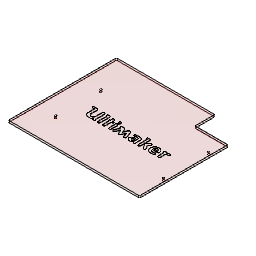
PCBCover_v9 (Autodesk Fusion 360 design; units mm, degrees)
Autodesk Fusion 360 part; units mm, degrees
note: some values were not read from the file. Set by a fixed rule: which sketch regions a step uses.
(part 1 of 5)
sketch "Sketch1" plane through (0, 0, 0) normal (0, 0, 1) x (1, 0, 0) in component "PCB Cover"
  line L0 (0, 0) -> (200, 0)
  line L1 (200, 0) -> (200, 165)
  line L2 (200, 165) -> (0, 165)
  line L3 (0, 165) -> (0, 0)
  line L4 (0, 42) -> (200, 42) construction
  line L5 (0, 111) -> (200, 111) construction
  line L6 (195, 165) -> (195, 0) construction
  line L7 (30, 165) -> (30, 0) construction
  circle A0 centre (30, 111) radius 1.5
  circle A1 centre (30, 42) radius 1.5
  circle A2 centre (195, 111) radius 1.5
  circle A3 centre (195, 42) radius 1.5
  line L8 (150, 165) -> (150, 135)
  line L9 (150, 135) -> (200, 135)
  dimension "d1_1" = 200
  dimension "d2_1" = 165
  dimension "d3_1" = 42
  dimension "d4_1" = 69
  dimension "d5_1" = 5
  dimension "d6_1" = 165
  dimension "d8_1" = 3
  dimension "d9_1" = 3
  dimension "d10_1" = 3
  dimension "d11_1" = 3
  dimension "d19" = 50
  dimension "d20" = 30
  constraint horizontal L0
  constraint vertical L1
  constraint horizontal L2
  constraint vertical L3
  constraint coincident L0.start L3.end
  constraint coincident L3 L4.start
  constraint coincident L1 L4.end
  constraint perpendicular L1 L4
  constraint coincident L3 L5.start
  constraint coincident L1 L5.end
  constraint perpendicular L1 L5
  constraint coincident L2 L6.start
  constraint coincident L0 L6.end
  constraint perpendicular L0 L6
  constraint coincident L2 L7.start
  constraint coincident L0 L7.end
  constraint perpendicular L0 L7
  constraint coincident L7 A0.centre
  constraint coincident L5 A0.centre
  constraint coincident L4 A1.centre
  constraint coincident L7 A1.centre
  constraint coincident L5 A2.centre
  constraint coincident L6 A2.centre
  constraint coincident L6 A3.centre
  constraint coincident L4 A3.centre
  constraint coincident L2 L8.start
  constraint perpendicular L2 L8
  constraint coincident L1 L9.end
  constraint perpendicular L1 L9
  measures "d1_1" distance of L1 L3
  measures "d2_1" distance of L0 L2
  measures "d3_1" distance of L0 L4
  measures "d4_1" distance of L4 L5
  measures "d5_1" distance of L1 L6
  measures "d6_1" distance of L6 L7
  measures "d8_1" diameter of A0
  measures "d9_1" diameter of A2
  measures "d10_1" diameter of A1
  measures "d11_1" diameter of A3
  measures "d19" distance of L1 L8
  measures "d20" distance of L2 L9
extrude "Extrude1" add sketch "Sketch1" along normal blind 3 contours L0 L1 L2 L3 L8 L9 in component "PCB Cover"
fillet "Fillet1" radius 1 6 edges at (0, 0, 1.5) (200, 0, 1.5) (0, 165, 1.5) (150, 165, 1.5) (150, 135, 1.5) (200, 135, 1.5) in component "PCB Cover"
sketch "Sketch3" plane through (0, 0, 3) normal (0, 0, 1) x (-1, 0, 0) in component "PCB Cover"
  arc A0 (-1, -165) -> (0, -164) centre (-1, -164) ccw
  line L0 (0, -164) -> (0, -1)
  arc A1 (0, -1) -> (-1, 0) centre (-1, -1) ccw
  line L1 (-1, 0) -> (-199, 0)
  arc A2 (-199, 0) -> (-200, -1) centre (-199, -1) ccw
  line L2 (-200, -1) -> (-200, -134)
  line L3 (-149, -165) -> (-1, -165)
  circle A3 centre (-195, -111) radius 1.5
  circle A4 centre (-195, -42) radius 1.5
  circle A5 centre (-30, -42) radius 1.5
  circle A6 centre (-30, -111) radius 1.5
  line L4 (-68.801, -83.1029) -> (-68.7045, -83.0443)
  line L5 (-134.3507, -66.6361) -> (-134.3896, -66.8178)
  line L6 (-62.8852, -66.514) -> (-62.9029, -66.3979)
  line L7 (-121.6987, -75.685) -> (-122.1036, -75.6545)
  line L8 (-118.5, -69.5598) -> (-118.5454, -69.7228)
  line L9 (-141.8993, -76.7576) -> (-141.9093, -76.9708)
  line L10 (-88.7696, -78.5031) -> (-88.9694, -78.4589)
  line L11 (-89.0089, -83.178) -> (-89.1669, -83.1019)
  line L12 (-112.6227, -67.3536) -> (-112.6072, -67.5226)
  line L13 (-88.9694, -78.4589) -> (-89.1489, -78.3988)
  line L14 (-122.1036, -75.6545) -> (-122.294, -75.6283)
  line L15 (-129.3707, -81.8373) -> (-129.3995, -81.725)
  line L16 (-79.0047, -82.0756) -> (-78.8216, -82.0548)
  line L17 (-130.9813, -66.8178) -> (-131.0201, -66.6361)
  line L18 (-62.9029, -66.3979) -> (-62.9317, -66.2857)
  line L19 (-93.4282, -77.1585) -> (-93.4342, -77.0387)
  line L20 (-141.7632, -77.5869) -> (-141.6868, -77.7243)
  line L21 (-129.7727, -81.1699) -> (-129.8628, -81.1025)
  line L22 (-90.112, -81.5125) -> (-90.103, -81.3276)
  line L23 (-76.2839, -77.4043) -> (-76.2551, -77.2923)
  line L24 (-69.6946, -66.6366) -> (-69.7482, -66.468)
  line L25 (-118.4981, -68.9082) -> (-118.4726, -69.0494)
  line L26 (-52.3978, -83.2329) -> (-52.2486, -83.2445)
  line L27 (-108.4802, -77.8696) -> (-108.3282, -77.9669)
  line L28 (-73.0643, -66.8183) -> (-73.088, -67.0129)
  line L29 (-109.5517, -66.2313) -> (-109.6365, -66.1302)
  line L30 (-98.0467, -78.3289) -> (-94.5986, -78.3289)
  line L31 (-117.5374, -72.5382) -> (-117.3342, -72.4627)
  line L32 (-54.1692, -81.8436) -> (-54.1178, -82.0155)
  line L33 (-120.6684, -72.9315) -> (-120.5332, -72.9709)
  line L34 (-156.7744, -71.3956) -> (-156.9307, -71.4261)
  line L35 (-135.3769, -72.8016) -> (-135.4061, -72.608)
  line L36 (-102.0665, -65.767) -> (-102.0887, -65.7551)
  line L37 (-101.3094, -66.4135) -> (-101.3514, -66.355)
  line L38 (-130.1691, -83.1912) -> (-130.0616, -83.1518)
  line L39 (-77.8285, -81.5268) -> (-77.7337, -81.3976)
  line L40 (-68.5313, -81.246) -> (-68.6144, -81.1705)
  line L41 (-134.1478, -82.5385) -> (-134.053, -82.6678)
  line L42 (-93.9443, -76.1877) -> (-94.0408, -76.1291)
  line L43 (-131.425, -65.9244) -> (-131.5448, -65.8219)
  line L44 (-65.2234, -72.2146) -> (-65.2234, -81.2746)
  line L45 (-109.0017, -77.3755) -> (-108.8856, -77.5138)
  line L46 (-98.1858, -78.3189) -> (-98.0467, -78.3289)
  line L47 (-73.0304, -82.0535) -> (-72.9802, -82.2175)
  line L48 (-121.4694, -71.7956) -> (-121.4581, -71.9616)
  line L49 (-133.6942, -65.7328) -> (-133.8257, -65.8219)
  line L50 (-70.2196, -65.8224) -> (-70.3511, -65.7333)
  line L51 (-59.741, -68.9094) -> (-59.5923, -68.8427)
  line L52 (-104.0125, -66.1757) -> (-104.086, -66.2611)
  line L53 (-86.5793, -82.05) -> (-86.64, -82.2161)
  line L54 (-93.6955, -76.4137) -> (-93.7711, -76.3306)
  line L55 (-53.0837, -83.0778) -> (-52.9126, -83.1337)
  line L56 (-110.7765, -65.5715) -> (-110.908, -65.5665)
  line L57 (-62.6523, -83.1446) -> (-62.4675, -83.0838)
  line L58 (-87.1608, -65.7896) -> (-87.0368, -65.8914)
  line L59 (-129.3707, -82.3092) -> (-129.353, -82.193)
  line L60 (-99.6212, -77.9746) -> (-99.4654, -78.0571)
  line L61 (-132.3759, -83.2437) -> (-130.5171, -83.2437)
  line L62 (-87.2947, -80.0143) -> (-87.1556, -80.1182)
  line L63 (-135.417, -73.5132) -> (-135.39, -73.3534)
  line L64 (-78.3302, -81.9099) -> (-78.1873, -81.8343)
  line L65 (-166.0715, -78.5875) -> (-165.9299, -78.5695)
  line L66 (-86.6139, -77.3087) -> (-86.6505, -77.4665)
  line L67 (-102.4573, -65.6498) -> (-102.6019, -65.6294)
  line L68 (-88.1205, -79.7153) -> (-87.941, -79.7427)
  line L69 (-92.9842, -66.7) -> (-93.0475, -66.548)
  line L70 (-54.9561, -69.5643) -> (-54.859, -69.6851)
  line L71 (-61.6272, -82.4034) -> (-61.5365, -82.243)
  line L72 (-61.4612, -82.0706) -> (-61.4018, -81.887)
  line L73 (-135.5106, -72.2342) -> (-135.5805, -72.0567)
  line L74 (-110.2717, -65.6893) -> (-110.3937, -65.6458)
  line L75 (-87.3025, -78.3238) -> (-87.4627, -78.3988)
  line L76 (-73.0668, -81.8773) -> (-73.0304, -82.0535)
  line L77 (-98.4083, -78.3) -> (-98.3201, -78.293)
  line L78 (-86.7617, -77.7607) -> (-86.8381, -77.8951)
  line L79 (-86.8381, -77.8951) -> (-86.9295, -78.0196)
  line L80 (-109.7282, -66.0365) -> (-109.8263, -65.9506)
  line L81 (-69.0109, -80.9558) -> (-69.1231, -80.927)
  line L82 (-90.0311, -82.05) -> (-90.0756, -81.8768)
  line L83 (-135.3726, -73.1817) -> (-135.3666, -72.9978)
  line L84 (-69.624, -80.9033) -> (-69.624, -67.2204)
  line L85 (-138.937, -77.8736) -> (-135.9197, -74.5208)
  line L86 (-88.7696, -65.5214) -> (-88.5487, -65.4942)
  line L87 (-105.5984, -77.78) -> (-105.4645, -77.6658)
  line L88 (-129.4388, -81.6175) -> (-129.4881, -81.5151)
  line L89 (-93.0475, -66.548) -> (-93.125, -66.4027)
  line L90 (-50.3366, -72.2147) -> (-50.3446, -71.781)
  line L91 (-59.1098, -68.6816) -> (-58.937, -68.6408)
  line L92 (-76.4986, -77.8006) -> (-76.4312, -77.7105)
  line L93 (-112.2905, -66.2655) -> (-112.3816, -66.403)
  line L94 (-101.743, -65.9554) -> (-101.7987, -65.9127)
  line L95 (-55.5404, -69.0628) -> (-55.4106, -69.1495)
  line L96 (-166.2167, -78.5935) -> (-166.0715, -78.5875)
  line L97 (-139.2218, -78.1381) -> (-139.075, -78.0114)
  line L98 (-88.063, -65.4942) -> (-87.842, -65.5214)
  line L99 (-50.3446, -71.781) -> (-50.3698, -71.3623)
  line L100 (-117.2991, -65.7945) -> (-117.4702, -65.7305)
  line L101 (-135.7422, -74.2993) -> (-135.641, -74.1334)
  line L102 (-108.7595, -77.6426) -> (-108.6242, -77.7613)
  line L103 (-168.7068, -75.6501) -> (-168.8644, -75.6788)
  line L104 (-89.0089, -79.8479) -> (-88.8429, -79.7872)
  line L105 (-66.3009, -66.1782) -> (-66.3403, -66.2857)
  line L106 (-46.1692, -81.9544) -> (-46.187, -81.8381)
  line L107 (-134.3896, -66.8178) -> (-134.4133, -67.0124)
  line L108 (-80.6588, -81.3976) -> (-80.5641, -81.5268)
  line L109 (-65.5702, -67.7507) -> (-65.458, -67.7795)
  line L110 (-101.9294, -65.8342) -> (-102.0665, -65.767)
  line L111 (-118.4726, -69.0494) -> (-118.4636, -69.1947)
  line L112 (-105.1182, -77.267) -> (-105.0233, -77.1168)
  line L113 (-46.5062, -81.2463) -> (-46.5893, -81.1708)
  line L114 (-109.2926, -66.7055) -> (-109.3443, -66.577)
  line L115 (-103.256, -65.7012) -> (-103.3662, -65.7391)
  line L116 (-73.096, -67.2204) -> (-73.096, -81.4885)
  line L117 (-46.5062, -82.9017) -> (-46.4306, -82.8186)
  line L118 (-65.7801, -67.6622) -> (-65.6778, -67.7114)
  line L119 (-66.2516, -67.1913) -> (-66.1929, -67.2877)
  line L120 (-86.5744, -67.0481) -> (-86.5694, -67.2203)
  line L121 (-76.4312, -77.7105) -> (-76.3726, -77.614)
  line L122 (-76.2551, -77.2923) -> (-76.2374, -77.1762)
  line L123 (-133.2339, -83.1617) -> (-133.0602, -83.1964)
  line L124 (-94.9876, -65.6109) -> (-95.1128, -65.6452)
  line L125 (-72.8225, -66.17) -> (-72.904, -66.3124)
  line L126 (-62.2947, -83.007) -> (-62.1343, -82.9148)
  line L127 (-80.4565, -65.8538) -> (-80.564, -65.9697)
  line L128 (-80.3368, -65.7513) -> (-80.4565, -65.8538)
  line L129 (-68.7045, -83.0443) -> (-68.6144, -82.9769)
  line L130 (-61.2891, -71.2837) -> (-61.2627, -71.0913)
  line L131 (-103.4191, -65.7552) -> (-103.4417, -65.7676)
  line L132 (-129.7727, -82.9765) -> (-129.6896, -82.9009)
  line L133 (-89.6998, -80.3631) -> (-89.5832, -80.2348)
  line L134 (-119.1134, -68.0951) -> (-118.9816, -68.1873)
  line L135 (-110.0394, -65.803) -> (-110.1534, -65.7418)
  line L136 (-107.288, -78.2938) -> (-107.0996, -78.3008)
  line L137 (-66.1929, -67.2877) -> (-66.1255, -67.3777)
  line L138 (-107.0926, -78.3) -> (-106.9084, -78.293)
  line L139 (-79.3885, -82.0756) -> (-79.1967, -82.0826)
  line L140 (-61.3587, -81.6928) -> (-61.3325, -81.4884)
  line L141 (-95.5765, -65.8721) -> (-95.6805, -65.95)
  line L142 (-86.6995, -66.407) -> (-86.6505, -66.5581)
  line L143 (-56.1554, -65.4904) -> (-56.5461, -65.4465)
  line L144 (-64.0494, -65.4636) -> (-65.222, -65.4636)
  line L145 (-79.9088, -65.5246) -> (-80.0624, -65.5866)
  line L146 (-65.8766, -65.6634) -> (-65.9667, -65.7308)
  line L147 (-66.3868, -66.7532) -> (-66.3691, -66.8694)
  line L148 (-80.5641, -81.5268) -> (-80.4566, -81.6427)
  line L149 (-80.8617, -80.931) -> (-80.8081, -81.0996)
  line L150 (-73.088, -67.0129) -> (-73.096, -67.2204)
  line L151 (-118.8637, -68.2887) -> (-118.7602, -68.3986)
  line L152 (-86.5074, -81.3276) -> (-86.4984, -81.5125)
  line L153 (-93.4519, -76.9224) -> (-93.4808, -76.8102)
  line L154 (-79.1967, -82.0826) -> (-79.0047, -82.0756)
  line L155 (-68.2409, -81.7256) -> (-68.2803, -81.618)
  line L156 (-136.1478, -71.1145) -> (-136.2972, -70.9305)
  line L157 (-129.6896, -81.2454) -> (-129.7727, -81.1699)
  line L158 (-78.8213, -65.4417) -> (-79.0043, -65.4208)
  line L159 (-101.7987, -65.9127) -> (-101.9294, -65.8342)
  line L160 (-93.9443, -78.129) -> (-93.8542, -78.0616)
  line L161 (-133.6942, -82.9756) -> (-133.5514, -83.0512)
  line L162 (-141.8251, -76.4251) -> (-141.8708, -76.5779)
  line L163 (-157.3994, -71.6624) -> (-157.4807, -71.7542)
  line L164 (-116.1043, -71.7474) -> (-115.9599, -71.6151)
  line L165 (-80.8617, -66.5655) -> (-80.9006, -66.7472)
  line L166 (-76.3233, -76.6007) -> (-76.3726, -76.4984)
  line L167 (-94.479, -78.3229) -> (-94.3628, -78.3051)
  line L168 (-140.2687, -78.5396) -> (-140.0758, -78.5266)
  line L169 (-55.9677, -68.8427) -> (-55.8191, -68.9094)
  line L170 (-80.9323, -78.2305) -> (-80.9323, -80.3472)
  line L171 (-109.4051, -66.455) -> (-109.4744, -66.3396)
  line L172 (-86.5348, -81.8768) -> (-86.5793, -82.05)
  line L173 (-118.5454, -69.7228) -> (-118.6087, -69.8735)
  line L174 (-159.5765, -77.2694) -> (-159.5942, -77.1532)
  line L175 (-94.8598, -65.586) -> (-94.9876, -65.6109)
  line L176 (-135.8309, -74.4188) -> (-135.7422, -74.2993)
  line L177 (-141.1482, -65.4851) -> (-141.3194, -65.4941)
  line L178 (-72.9166, -82.3692) -> (-72.8402, -82.5087)
  line L179 (-160.5044, -78.5352) -> (-160.3923, -78.5064)
  line L180 (-110.3937, -65.6458) -> (-110.5188, -65.6115)
  line L181 (-63.2738, -83.2247) -> (-63.056, -83.2157)
  line L182 (-165.6589, -78.5) -> (-165.5305, -78.4495)
  line L183 (-126.9226, -75.2022) -> (-126.9006, -75.4218)
  line L184 (-165.5305, -78.4495) -> (-165.4074, -78.3891)
  line L185 (-65.6778, -67.7114) -> (-65.5702, -67.7507)
  line L186 (-62.9711, -66.1782) -> (-63.0204, -66.076)
  line L187 (-76.3233, -77.5118) -> (-76.2839, -77.4043)
  line L188 (-59.4375, -68.7825) -> (-59.2767, -68.7288)
  line L189 (-80.9243, -66.9418) -> (-80.9323, -67.1493)
  line L190 (-59.6322, -65.5243) -> (-59.9762, -65.5837)
  line L191 (-120.4347, -70.8642) -> (-120.6989, -70.9072)
  line L192 (-106.9084, -78.293) -> (-106.7273, -78.2719)
  line L193 (-140.1409, -65.7466) -> (-140.2391, -65.691)
  line L194 (-83.5412, -77.2401) -> (-83.5221, -77.3781)
  line L195 (-161.4459, -66.1697) -> (-161.5406, -66.0405)
  line L196 (-89.912, -77.6175) -> (-89.961, -77.4665)
  line L197 (-123.9451, -66.3953) -> (-124.0398, -66.2386)
  line L198 (-118.9041, -70.2565) -> (-119.0371, -70.363)
  line L199 (-102.3649, -65.6702) -> (-102.4573, -65.6498)
  line L200 (-127.2707, -67.0128) -> (-127.2303, -67.206)
  line L201 (-122.801, -75.494) -> (-122.9443, -75.4272)
  line L202 (-95.3531, -65.7412) -> (-95.4672, -65.8024)
  line L203 (-148.3368, -72.1199) -> (-148.3504, -72.4808)
  line L204 (-88.5487, -65.4942) -> (-88.3059, -65.4852)
  line L205 (-142.7808, -67.0086) -> (-142.7888, -67.1725)
  line L206 (-54.237, -81.2746) -> (-54.229, -81.4727)
  line L207 (-156.082, -76.7687) -> (-155.8755, -76.964)
  line L208 (-131.0201, -66.6361) -> (-131.0736, -66.4674)
  line L209 (-118.5979, -68.6408) -> (-118.54, -68.7717)
  line L210 (-72.9718, -66.468) -> (-73.0254, -66.6366)
  line L211 (-83.1465, -77.9726) -> (-83.0413, -78.0357)
  line L212 (-140.5788, -65.5579) -> (-140.708, -65.5271)
  line L213 (-160.7403, -76.2193) -> (-161.1724, -76.2193)
  line L214 (-163.2831, -65.5128) -> (-163.4568, -65.5474)
  line L215 (-159.6623, -77.8448) -> (-159.623, -77.7373)
  line L216 (-125.5222, -77.3626) -> (-125.317, -77.4711)
  line L217 (-103.4417, -65.7676) -> (-103.5785, -65.8343)
  line L218 (-72.7513, -82.6359) -> (-72.6504, -82.7506)
  line L219 (-80.9006, -66.7472) -> (-80.9243, -66.9418)
  line L220 (-107.0996, -78.3008) -> (-107.0926, -78.3)
  line L221 (-131.1414, -66.3118) -> (-131.2229, -66.1694)
  line L222 (-159.623, -77.7373) -> (-159.5942, -77.6251)
  line L223 (-115.5046, -67.2364) -> (-115.6051, -67.0878)
  line L224 (-105.0233, -77.1168) -> (-104.9397, -76.9586)
  line L225 (-69.0109, -83.1916) -> (-68.9034, -83.1522)
  line L226 (-87.4437, -83.1019) -> (-87.6017, -83.178)
  line L227 (-129.8628, -81.1025) -> (-129.9593, -81.0439)
  line L228 (-93.3205, -66.1366) -> (-93.4375, -66.0181)
  line L229 (-61.7328, -82.5514) -> (-61.6272, -82.4034)
  line L230 (-95.1128, -65.6452) -> (-95.2348, -65.6887)
  line L231 (-92.9022, -67.0198) -> (-92.9356, -66.8576)
  line L232 (-65.3418, -67.7972) -> (-65.2235, -67.8035)
  line L233 (-125.4473, -65.4949) -> (-125.7165, -65.4841)
  line L234 (-89.8498, -77.7607) -> (-89.912, -77.6175)
  line L235 (-135.4521, -73.6609) -> (-135.417, -73.5132)
  line L236 (-54.859, -69.6851) -> (-54.7687, -69.813)
  line L237 (-80.8081, -81.0996) -> (-80.7403, -81.2552)
  line L238 (-159.623, -77.0411) -> (-159.6623, -76.9336)
  line L239 (-141.7635, -76.2923) -> (-141.8251, -76.4251)
  line L240 (-53.5344, -82.8302) -> (-53.395, -82.9256)
  line L241 (-142.3164, -65.9988) -> (-142.4212, -66.1208)
  line L242 (-87.6017, -83.178) -> (-87.7677, -83.2388)
  line L243 (-145.3418, -69.2555) -> (-145.4536, -68.9872)
  line L244 (-101.1722, -66.6714) -> (-101.2359, -66.5385)
  line L245 (-94.0408, -78.1876) -> (-93.9443, -78.129)
  line L246 (-116.2139, -66.4357) -> (-116.3544, -66.3241)
  line L247 (-134.4213, -81.4877) -> (-134.4133, -81.6953)
  line L248 (-54.0527, -82.1779) -> (-53.9742, -82.3302)
  line L249 (-159.5765, -77.5088) -> (-159.5705, -77.3891)
  line L250 (-87.0272, -80.2348) -> (-86.9106, -80.3631)
  line L251 (-106.7273, -78.2719) -> (-106.5499, -78.2376)
  line L252 (-120.8684, -65.7284) -> (-121.1733, -65.8221)
  line L253 (-46.5893, -82.9773) -> (-46.5062, -82.9017)
  line L254 (-145.8673, -68.2144) -> (-146.032, -67.9697)
  line L255 (-76.3726, -77.614) -> (-76.3233, -77.5118)
  line L256 (-132.6853, -65.4846) -> (-132.8771, -65.4916)
  line L257 (-72.0727, -65.5958) -> (-72.2263, -65.6578)
  line L258 (-114.9918, -69.0276) -> (-114.9978, -68.8249)
  line L259 (-64.2526, -83.007) -> (-64.0798, -83.0838)
  line L260 (-58.1882, -68.5413) -> (-57.78, -68.5289)
  line L261 (-89.961, -77.4665) -> (-89.9976, -77.3087)
  line L262 (-129.5467, -81.4186) -> (-129.6141, -81.3285)
  line L263 (-55.1702, -69.3433) -> (-55.0598, -69.4503)
  line L264 (-134.4213, -67.22) -> (-134.4213, -69.8591)
  line L265 (-119.5881, -67.881) -> (-119.417, -67.9412)
  line L266 (-104.1992, -66.4149) -> (-104.2726, -66.5393)
  line L267 (-159.996, -78.2921) -> (-159.9129, -78.2166)
  line L268 (-83.5412, -76.9402) -> (-83.5472, -77.0903)
  line L269 (-63.056, -83.2157) -> (-62.8487, -83.1888)
  line L270 (-54.2713, -71.2837) -> (-54.2524, -71.4835)
  line L271 (-83.3207, -77.8168) -> (-83.2396, -77.8997)
  line L272 (-164.9783, -78.0585) -> (-164.8891, -77.9561)
  line L273 (-77.936, -81.6427) -> (-77.8285, -81.5268)
  line L274 (-164.4235, -77.7499) -> (-164.3546, -77.8655)
  line L275 (-80.564, -65.9697) -> (-80.6588, -66.0989)
  line L276 (-161.1724, -76.2193) -> (-161.1724, -67.2203)
  line L277 (-163.2193, -78.5212) -> (-163.0667, -78.5355)
  line L278 (-119.0371, -70.363) -> (-119.1872, -70.4597)
  line L279 (-130.0616, -83.1518) -> (-129.9593, -83.1025)
  line L280 (-80.2054, -81.8343) -> (-80.0626, -81.9099)
  line L281 (-119.1872, -70.4597) -> (-119.354, -70.5472)
  line L282 (-127.1583, -66.2762) -> (-127.213, -66.401)
  line L283 (-107.8316, -78.1881) -> (-107.6547, -78.2368)
  line L284 (-157.4807, -71.7542) -> (-157.549, -71.8607)
  line L285 (-161.1724, -67.2203) -> (-161.1804, -67.0127)
  line L286 (-46.3632, -81.4195) -> (-46.4306, -81.3294)
  line L287 (-93.8542, -76.2551) -> (-93.9443, -76.1877)
  line L288 (-46.6794, -83.0447) -> (-46.5893, -82.9773)
  line L289 (-146.6097, -67.2837) -> (-146.8308, -67.0731)
  line L290 (-99.3035, -78.1282) -> (-99.1359, -78.1876)
  line L291 (-46.1632, -82.0741) -> (-46.1692, -81.9544)
  line L292 (-83.2396, -77.8997) -> (-83.1465, -77.9726)
  line L293 (-79.909, -81.9719) -> (-79.7451, -82.0202)
  line L294 (-135.9197, -74.5208) -> (-135.8309, -74.4188)
  line L295 (-164.808, -77.8468) -> (-164.7355, -77.7311)
  line L296 (-61.2576, -65.9312) -> (-61.5536, -66.0458)
  line L297 (-102.7545, -71.7649) -> (-100.6403, -76.7941)
  line L298 (-89.9976, -77.3087) -> (-90.0226, -77.145)
  line L299 (-103.3662, -65.7391) -> (-103.4191, -65.7552)
  line L300 (-133.9455, -82.7838) -> (-133.8257, -82.8864)
  line L301 (-65.2235, -67.8035) -> (-65.2215, -71.648)
  line L302 (-161.3644, -66.3121) -> (-161.4459, -66.1697)
  line L303 (-94.5986, -78.3289) -> (-94.479, -78.3229)
  line L304 (-68.1943, -81.9542) -> (-68.2121, -81.8379)
  line L305 (-68.9034, -80.9952) -> (-69.0109, -80.9558)
  line L306 (-82.9243, -78.0894) -> (-82.7955, -78.134)
  line L307 (-94.3628, -76.0117) -> (-94.479, -75.994)
  line L308 (-160.1826, -78.4179) -> (-160.0861, -78.3594)
  line L309 (-103.7091, -65.9129) -> (-103.7659, -65.9563)
  line L310 (-164.5739, -66.6363) -> (-164.6128, -66.8181)
  line L311 (-164.6183, -77.4824) -> (-164.5745, -77.3505)
  line L312 (-65.458, -65.4873) -> (-65.5702, -65.5161)
  line L313 (-79.5712, -65.4417) -> (-79.7449, -65.4763)
  line L314 (-122.1871, -78.2057) -> (-121.4511, -78.2582)
  line L315 (-94.1431, -78.2369) -> (-94.0408, -78.1876)
  line L316 (-83.0413, -78.0357) -> (-82.9243, -78.0894)
  line L317 (-151.4448, -78.5402) -> (-151.064, -78.5322)
  line L318 (-164.6445, -74.2229) -> (-166.4853, -75.6143)
  line L319 (-80.9323, -80.3472) -> (-80.9243, -80.5547)
  line L320 (-163.6208, -65.5957) -> (-163.7744, -65.6576)
  line L321 (-100.1696, -77.5402) -> (-100.045, -77.6636)
  line L322 (-105.8898, -77.9776) -> (-105.7403, -77.8841)
  line L323 (-53.9742, -82.3302) -> (-53.8827, -82.4721)
  line L324 (-119.2563, -65.4903) -> (-119.5906, -65.5093)
  line L325 (-159.8374, -78.1336) -> (-159.7701, -78.0436)
  line L326 (-161.2966, -66.4677) -> (-161.3644, -66.3121)
  line L327 (-126.9332, -68.8866) -> (-126.9296, -69.1468)
  line L328 (-93.4808, -76.8102) -> (-93.5202, -76.7026)
  line L329 (-57.78, -68.5289) -> (-57.3718, -68.5413)
  line L330 (-63.4915, -83.2157) -> (-63.2738, -83.2247)
  line L331 (-94.0212, -65.666) -> (-94.1649, -65.6216)
  line L332 (-69.7482, -66.468) -> (-69.816, -66.3124)
  line L333 (-95.9551, -66.2307) -> (-96.0325, -66.3391)
  line L334 (-93.125, -66.4027) -> (-93.2162, -66.2652)
  line L335 (-118.7602, -68.3986) -> (-118.6715, -68.5162)
  line L336 (-119.417, -67.9412) -> (-119.2587, -68.0128)
  line L337 (-77.4682, -80.5547) -> (-77.4602, -80.3472)
  line L338 (-54.4764, -70.3947) -> (-54.4209, -70.5579)
  line L339 (-123.4576, -70.2886) -> (-123.444, -70.0488)
  line L340 (-164.5203, -66.4677) -> (-164.5739, -66.6363)
  line L341 (-57.7791, -65.3904) -> (-58.167, -65.3954)
  line L342 (-161.7678, -65.8222) -> (-161.8993, -65.7331)
  line L343 (-159.7701, -78.0436) -> (-159.7115, -77.9471)
  line L344 (-159.5942, -77.6251) -> (-159.5765, -77.5088)
  line L345 (-129.5467, -82.7277) -> (-129.4881, -82.6312)
  line L346 (-53.2446, -83.0083) -> (-53.0837, -83.0778)
  line L347 (-82.5031, -78.1971) -> (-82.3396, -78.2162)
  line L348 (-116.0463, -77.5203) -> (-115.9387, -77.4488)
  line L349 (-95.7786, -66.0359) -> (-95.8703, -66.1296)
  line L350 (-161.2041, -66.8181) -> (-161.243, -66.6363)
  line L351 (-165.0752, -78.1535) -> (-164.9783, -78.0585)
  line L352 (-109.4744, -66.3396) -> (-109.5517, -66.2313)
  line L353 (-142.2007, -65.8871) -> (-142.3164, -65.9988)
  line L354 (-104.868, -76.793) -> (-102.7545, -71.7649)
  line L355 (-161.1804, -67.0127) -> (-161.2041, -66.8181)
  line L356 (-76.7473, -76.0857) -> (-76.8438, -76.0271)
  line L357 (-162.3596, -65.5474) -> (-162.5333, -65.5128)
  line L358 (-46.9857, -83.192) -> (-46.8782, -83.1526)
  line L359 (-130.5171, -83.2437) -> (-130.3974, -83.2377)
  line L360 (-87.941, -83.2833) -> (-88.1205, -83.3107)
  line L361 (-68.4557, -81.3291) -> (-68.5313, -81.246)
  line L362 (-64.9198, -82.4034) -> (-64.8142, -82.5514)
  line L363 (-145.7175, -75.4276) -> (-145.5747, -75.1445)
  line L364 (-125.2007, -65.5269) -> (-125.4473, -65.4949)
  line L365 (-98.4224, -78.299) -> (-98.4083, -78.3)
  line L366 (-131.0736, -66.4674) -> (-131.1414, -66.3118)
  line L367 (-133.3978, -65.5954) -> (-133.5514, -65.6573)
  line L368 (-104.9397, -76.9586) -> (-104.868, -76.793)
  line L369 (-124.4241, -65.8412) -> (-124.5884, -65.7372)
  line L370 (-98.7865, -78.2694) -> (-98.606, -78.291)
  line L371 (-77.4016, -75.8859) -> (-77.4602, -75.8859)
  line L372 (-47.0979, -83.2208) -> (-46.9857, -83.192)
  line L373 (-88.9694, -65.5656) -> (-88.7696, -65.5214)
  line L374 (-164.6128, -66.8181) -> (-164.6365, -67.0127)
  line L375 (-163.9172, -65.7331) -> (-164.0488, -65.8222)
  line L376 (-111.3423, -65.6222) -> (-111.4862, -65.6666)
  line L377 (-164.6445, -69.8598) -> (-164.6445, -73.5928)
  line L378 (-164.7355, -77.7311) -> (-164.6721, -77.6095)
  line L379 (-89.9704, -80.809) -> (-89.8943, -80.6511)
  line L380 (-164.2761, -66.0405) -> (-164.3709, -66.1697)
  line L381 (-164.0488, -65.8222) -> (-164.1686, -65.9247)
  line L382 (-120.2483, -75.693) -> (-121.2699, -75.693)
  line L383 (-46.7759, -83.1033) -> (-46.6794, -83.0447)
  line L384 (-60.6361, -65.7353) -> (-60.9517, -65.8277)
  line L385 (-87.4627, -78.3988) -> (-87.6422, -78.4589)
  line L386 (-71.9818, -83.1371) -> (-71.8185, -83.1765)
  line L387 (-122.887, -66.7624) -> (-123.1539, -66.9883)
  line L388 (-119.3494, -72.958) -> (-118.8696, -72.8798)
  line L389 (-115.7616, -75.4972) -> (-115.8534, -75.4086)
  line L390 (-129.3995, -81.725) -> (-129.4388, -81.6175)
  line L391 (-64.4129, -82.9148) -> (-64.2526, -83.007)
  line L392 (-54.4209, -70.5579) -> (-54.3726, -70.7284)
  line L393 (-72.538, -82.853) -> (-72.4145, -82.9429)
  line L394 (-134.3507, -82.0716) -> (-134.2971, -82.2404)
  line L395 (-133.0602, -83.1964) -> (-132.8771, -83.2173)
  line L396 (-99.7701, -77.8812) -> (-99.6212, -77.9746)
  line L397 (-139.7112, -78.4291) -> (-139.5402, -78.3492)
  line L398 (-105.3395, -77.542) -> (-105.2238, -77.4089)
  line L399 (-94.2506, -76.0405) -> (-94.3628, -76.0117)
  line L400 (-162.5333, -65.5128) -> (-162.7163, -65.4919)
  line L401 (-168.5423, -78.5586) -> (-168.3718, -78.5846)
  line L402 (-109.3525, -76.7362) -> (-109.2832, -76.9079)
  line L403 (-130.2812, -80.9265) -> (-130.3974, -80.9088)
  line L404 (-55.4058, -65.6166) -> (-55.7752, -65.5471)
  line L405 (-132.3103, -65.5125) -> (-132.4933, -65.4916)
  line L406 (-161.243, -66.6363) -> (-161.2966, -66.4677)
  line L407 (-123.444, -70.0488) -> (-123.4038, -69.8118)
  line L408 (-126.7009, -65.772) -> (-126.8138, -65.8554)
  line L409 (-168.1963, -75.6143) -> (-168.3718, -75.6183)
  line L410 (-168.5423, -75.63) -> (-168.7068, -75.6501)
  line L411 (-127.1076, -67.6416) -> (-127.0421, -67.9152)
  line L412 (-89.8943, -82.3741) -> (-89.9704, -82.2161)
  line L413 (-140.5646, -78.5082) -> (-140.4165, -78.5316)
  line L414 (-116.5871, -72.0968) -> (-116.4183, -71.9879)
  line L415 (-118.7311, -65.4883) -> (-118.916, -65.4843)
  line L416 (-169.1558, -75.7645) -> (-169.2879, -75.8224)
  line L417 (-54.2977, -71.0913) -> (-54.2713, -71.2837)
  line L418 (-147.56, -77.4693) -> (-147.3075, -77.2905)
  line L419 (-163.4568, -65.5474) -> (-163.6208, -65.5957)
  line L420 (-156.4497, -68.5385) -> (-156.3519, -68.6121)
  line L421 (-83.4904, -77.5044) -> (-83.4462, -77.6194)
  line L422 (-89.5747, -65.8914) -> (-89.4507, -65.7896)
  line L423 (-130.5171, -80.9028) -> (-130.9496, -80.9028)
  line L424 (-51.1477, -68.5458) -> (-51.3135, -68.2591)
  line L425 (-149.6412, -78.3469) -> (-149.3113, -78.2634)
  line L426 (-120.5577, -65.6509) -> (-120.8684, -65.7284)
  line L427 (-104.3357, -66.6717) -> (-104.3427, -66.6878)
  line L428 (-168.7068, -78.5163) -> (-168.5423, -78.5586)
  line L429 (-163.7744, -65.6576) -> (-163.9172, -65.7331)
  line L430 (-159.9129, -78.2166) -> (-159.8374, -78.1336)
  line L431 (-164.6445, -73.5928) -> (-164.6445, -74.2229)
  line L432 (-165.1793, -78.2406) -> (-165.0752, -78.1535)
  line L433 (-134.4213, -69.8591) -> (-134.4213, -73.5926)
  line L434 (-169.0144, -75.7168) -> (-169.1558, -75.7645)
  line L435 (-124.6208, -77.7524) -> (-124.3621, -77.832)
  line L436 (-169.7772, -77.5459) -> (-169.705, -77.6958)
  line L437 (-169.705, -77.6958) -> (-169.6191, -77.8372)
  line L438 (-121.4511, -78.2582) -> (-120.6654, -78.2888)
  line L439 (-164.1686, -65.9247) -> (-164.2761, -66.0405)
  line L440 (-168.3718, -75.6183) -> (-168.5423, -75.63)
  line L441 (-123.8053, -77.9707) -> (-123.5073, -78.0302)
  line L442 (-115.2109, -70.4382) -> (-115.1452, -70.2308)
  line L443 (-89.8943, -80.6511) -> (-89.8038, -80.5021)
  line L444 (-145.4536, -68.9872) -> (-145.5783, -68.7237)
  line L445 (-61.3235, -81.2746) -> (-61.3235, -71.9056)
  line L446 (-118.9816, -68.1873) -> (-118.8637, -68.2887)
  line L447 (-76.6572, -77.9592) -> (-76.5741, -77.8837)
  line L448 (-47.3337, -83.2445) -> (-47.2141, -83.2385)
  line L449 (-119.9188, -65.542) -> (-120.2412, -65.589)
  line L450 (-93.4342, -77.0387) -> (-93.4519, -76.9224)
  line L451 (-56.5461, -65.4465) -> (-56.9471, -65.4152)
  line L452 (-65.2234, -81.2746) -> (-65.2144, -81.4884)
  line L453 (-55.2872, -69.243) -> (-55.1702, -69.3433)
  line L454 (-87.4627, -65.6257) -> (-87.3025, -65.7007)
  line L455 (-142.6551, -67.8835) -> (-142.5973, -68.0144)
  line L456 (-118.6715, -68.5162) -> (-118.5979, -68.6408)
  line L457 (-119.2587, -68.0128) -> (-119.1134, -68.0951)
  line L458 (-122.9886, -68.9274) -> (-122.8244, -68.7308)
  line L459 (-169.2879, -75.8224) -> (-169.4097, -75.8909)
  line L460 (-103.8578, -66.0282) -> (-103.9455, -66.1069)
  line L461 (-83.4462, -77.6194) -> (-83.3896, -77.7235)
  line L462 (-62.8487, -83.1888) -> (-62.6523, -83.1446)
  line L463 (-169.4097, -78.0911) -> (-169.2879, -78.2018)
  line L464 (-169.705, -76.165) -> (-169.7772, -76.2808)
  line L465 (-100.285, -77.4076) -> (-100.1696, -77.5402)
  line L466 (-151.0533, -71.3283) -> (-155.7174, -71.3283)
  line L467 (-102.7543, -65.6214) -> (-102.7551, -65.6214)
  line L468 (-94.3628, -78.3051) -> (-94.2506, -78.2763)
  line L469 (-124.0902, -77.9047) -> (-123.8053, -77.9707)
  line L470 (-123.3375, -69.5795) -> (-123.2458, -69.3535)
  line L471 (-135.4516, -72.4184) -> (-135.5106, -72.2342)
  line L472 (-109.2012, -77.0721) -> (-109.1071, -77.2281)
  line L473 (-157.6493, -72.1214) -> (-157.6826, -72.2773)
  line L474 (-90.042, -76.8042) -> (-90.042, -67.2203)
  line L475 (-122.4278, -68.3793) -> (-122.1967, -68.2279)
  line L476 (-55.7752, -65.5471) -> (-56.1554, -65.4904)
  line L477 (-124.2785, -65.9603) -> (-124.4241, -65.8412)
  line L478 (-116.1605, -77.5843) -> (-116.0463, -77.5203)
  line L479 (-73.0254, -66.6366) -> (-73.0643, -66.8183)
  line L480 (-59.5923, -68.8427) -> (-59.4375, -68.7825)
  line L481 (-159.7115, -77.9471) -> (-159.6623, -77.8448)
  line L482 (-65.0858, -82.0706) -> (-65.0105, -82.243)
  line L483 (-102.7591, -65.6214) -> (-102.906, -65.6294)
  line L484 (-124.3621, -77.832) -> (-124.0902, -77.9047)
  line L485 (-54.7002, -65.7945) -> (-55.0473, -65.699)
  line L486 (-89.309, -78.3238) -> (-89.4507, -78.2349)
  line L487 (-98.606, -78.291) -> (-98.4224, -78.299)
  line L488 (-115.3276, -67.551) -> (-115.412, -67.3908)
  line L489 (-88.8429, -83.2388) -> (-89.0089, -83.178)
  line L490 (-104.2726, -66.5393) -> (-104.3357, -66.6717)
  line L491 (-93.8542, -78.0616) -> (-93.7711, -77.986)
  line L492 (-116.5003, -66.219) -> (-116.6513, -66.1205)
  line L493 (-68.1883, -82.0739) -> (-68.1943, -81.9542)
  line L494 (-129.3995, -82.4213) -> (-129.3707, -82.3092)
  line L495 (-105.7403, -77.8841) -> (-105.5984, -77.78)
  line L496 (-123.4576, -74.5459) -> (-123.4576, -71.6447)
  line L497 (-68.801, -81.0445) -> (-68.9034, -80.9952)
  line L498 (-54.6086, -70.0896) -> (-54.539, -70.2386)
  line L499 (-150.9298, -71.3363) -> (-151.0533, -71.3283)
  line L500 (-73.096, -81.4885) -> (-73.089, -81.689)
  line L501 (-66.0499, -67.4608) -> (-65.9667, -67.5363)
  line L502 (-133.5514, -65.6573) -> (-133.6942, -65.7328)
  line L503 (-141.5982, -76.0604) -> (-141.6874, -76.173)
  line L504 (-116.8071, -66.0287) -> (-116.9672, -65.9437)
  line L505 (-89.4549, -80.1182) -> (-89.3159, -80.0143)
  line L506 (-150.2093, -68.431) -> (-150.0636, -68.4918)
  line L507 (-125.8714, -65.4901) -> (-126.0231, -65.5089)
  line L508 (-135.4936, -73.7968) -> (-135.4521, -73.6609)
  line L509 (-86.7161, -82.3741) -> (-86.8066, -82.5231)
  line L510 (-126.6674, -76.2071) -> (-126.5733, -76.3809)
  line L511 (-126.4497, -65.6347) -> (-126.5793, -65.6983)
  line L512 (-115.4379, -76.172) -> (-115.4648, -76.0496)
  line L513 (-64.0798, -83.0838) -> (-63.895, -83.1446)
  line L514 (-93.6281, -76.5038) -> (-93.6955, -76.4137)
  line L515 (-130.9496, -80.9028) -> (-130.9496, -67.22)
  line L516 (-52.7317, -83.1755) -> (-52.5415, -83.2028)
  line L517 (-120.7384, -67.7832) -> (-120.3905, -67.7689)
  line L518 (-76.2551, -76.8206) -> (-76.2839, -76.7083)
  line L519 (-117.8209, -65.624) -> (-117.9999, -65.5818)
  line L520 (-99.4654, -78.0571) -> (-99.3035, -78.1282)
  line L521 (-117.3342, -72.4627) -> (-117.1373, -72.3811)
  line L522 (-109.2832, -76.9079) -> (-109.2012, -77.0721)
  line L523 (-65.222, -65.4636) -> (-65.3418, -65.4696)
  line L524 (-115.5928, -77.0817) -> (-115.5319, -76.9681)
  line L525 (-86.5348, -81.1482) -> (-86.5074, -81.3276)
  line L526 (-69.2394, -80.9093) -> (-69.3591, -80.9033)
  line L527 (-111.9405, -65.911) -> (-112.0694, -66.0184)
  line L528 (-86.6505, -66.5581) -> (-86.6139, -66.7159)
  line L529 (-115.5801, -71.1668) -> (-115.4725, -70.9992)
  line L530 (-168.8644, -75.6788) -> (-169.0144, -75.7168)
  line L531 (-129.9593, -81.0439) -> (-130.0616, -80.9946)
  line L532 (-124.9758, -65.5788) -> (-125.2007, -65.5269)
  line L533 (-46.3046, -82.632) -> (-46.2553, -82.5297)
  line L534 (-134.4133, -67.0124) -> (-134.4213, -67.22)
  line L535 (-134.2293, -82.396) -> (-134.1478, -82.5385)
  line L536 (-47.2141, -83.2385) -> (-47.0979, -83.2208)
  line L537 (-94.2506, -78.2763) -> (-94.1431, -78.2369)
  line L538 (-159.5705, -77.3891) -> (-159.5765, -77.2694)
  line L539 (-122.8727, -78.1301) -> (-122.1871, -78.2057)
  line L540 (-62.1152, -66.3088) -> (-62.3805, -66.4572)
  line L541 (-103.9455, -66.1069) -> (-104.0125, -66.1757)
  line L542 (-116.4183, -71.9879) -> (-116.2573, -71.8716)
  line L543 (-54.3726, -70.7284) -> (-54.3315, -70.9062)
  line L544 (-139.5402, -78.3492) -> (-139.3769, -78.2514)
  line L545 (-122.294, -75.6283) -> (-122.4745, -75.5935)
  line L546 (-115.7132, -66.9451) -> (-115.8284, -66.8085)
  line L547 (-62.4675, -83.0838) -> (-62.2947, -83.007)
  line L548 (-132.6852, -83.2248) -> (-132.6154, -83.2188)
  line L549 (-126.864, -75.6319) -> (-126.8129, -75.8328)
  line L550 (-124.8662, -77.6658) -> (-124.6208, -77.7524)
  line L551 (-109.1071, -77.2281) -> (-109.0017, -77.3755)
  line L552 (-126.5793, -65.6983) -> (-126.7009, -65.772)
  line L553 (-130.0616, -80.9946) -> (-130.1691, -80.9553)
  line L554 (-103.5785, -65.8343) -> (-103.7091, -65.9129)
  line L555 (-72.6203, -65.9249) -> (-72.7278, -66.0408)
  line L556 (-169.6191, -76.0618) -> (-169.705, -76.165)
  line L557 (-71.5521, -65.492) -> (-71.7351, -65.5129)
  line L558 (-66.3691, -66.3979) -> (-66.3868, -66.514)
  line L559 (-122.6372, -68.5476) -> (-122.4278, -68.3793)
  line L560 (-92.9356, -66.8576) -> (-92.9842, -66.7)
  line L561 (-86.64, -82.2161) -> (-86.7161, -82.3741)
  line L562 (-115.447, -76.7125) -> (-115.4247, -76.5699)
  line L563 (-112.459, -66.5484) -> (-112.5222, -66.7004)
  line L564 (-156.2767, -76.5651) -> (-156.082, -76.7687)
  line L565 (-141.8993, -77.1333) -> (-141.8708, -77.2907)
  line L566 (-104.086, -66.2611) -> (-104.1537, -66.3521)
  line L567 (-120.173, -67.7759) -> (-119.9665, -67.7976)
  line L568 (-111.6483, -65.734) -> (-111.7999, -65.8158)
  line L569 (-83.5221, -77.3781) -> (-83.4904, -77.5044)
  line L570 (-100.3903, -77.2662) -> (-100.285, -77.4076)
  line L571 (-66.1255, -67.3777) -> (-66.0499, -67.4608)
  line L572 (-142.5973, -68.0144) -> (-142.5381, -68.1262)
  line L573 (-52.5415, -83.2028) -> (-52.3978, -83.2329)
  line L574 (-89.8038, -80.5021) -> (-89.6998, -80.3631)
  line L575 (-126.8129, -75.8328) -> (-126.7473, -76.0244)
  line L576 (-134.2293, -66.3118) -> (-134.2971, -66.4674)
  line L577 (-118.8696, -72.8798) -> (-118.406, -72.7853)
  line L578 (-116.9469, -72.2931) -> (-116.7634, -72.1984)
  line L579 (-110.1534, -65.7418) -> (-110.2717, -65.6893)
  line L580 (-119.9037, -73.0252) -> (-119.8428, -73.0222)
  line L581 (-169.903, -77.0537) -> (-169.877, -77.2239)
  line L582 (-69.8975, -66.17) -> (-69.9923, -66.0408)
  line L583 (-127.2303, -67.206) -> (-127.1731, -67.4104)
  line L584 (-108.3282, -77.9669) -> (-108.169, -78.0527)
  line L585 (-135.5805, -72.0567) -> (-135.6585, -71.8872)
  line L586 (-62.8792, -66.6336) -> (-62.8852, -66.514)
  line L587 (-72.5006, -65.8224) -> (-72.6203, -65.9249)
  line L588 (-157.549, -71.8607) -> (-157.605, -71.9829)
  line L589 (-65.1452, -81.887) -> (-65.0858, -82.0706)
  line L590 (-157.605, -71.9829) -> (-157.6493, -72.1214)
  line L591 (-86.7617, -66.2638) -> (-86.6995, -66.407)
  line L592 (-120.4012, -72.9983) -> (-120.2756, -73.0155)
  line L593 (-72.2803, -83.0202) -> (-72.1359, -83.085)
  line L594 (-147.824, -77.6353) -> (-147.56, -77.4693)
  line L595 (-132.4975, -83.2377) -> (-132.3759, -83.2437)
  line L596 (-51.8966, -67.4839) -> (-52.1188, -67.2535)
  line L597 (-119.9665, -67.7976) -> (-119.7714, -67.8329)
  line L598 (-70.4939, -65.6578) -> (-70.6475, -65.5958)
  line L599 (-159.5942, -77.1532) -> (-159.623, -77.0411)
  line L600 (-115.6648, -77.1863) -> (-115.5928, -77.0817)
  line L601 (-89.5832, -82.7907) -> (-89.6998, -82.6623)
  line L602 (-100.4851, -77.1166) -> (-100.3903, -77.2662)
  line L603 (-168.8644, -78.4586) -> (-168.7068, -78.5163)
  line L604 (-109.3443, -66.577) -> (-109.4051, -66.455)
  line L605 (-168.3718, -78.5846) -> (-168.1962, -78.5935)
  line L606 (-126.3132, -65.5816) -> (-126.4497, -65.6347)
  line L607 (-65.7801, -65.6048) -> (-65.8766, -65.6634)
  line L608 (-114.9978, -69.2913) -> (-114.9918, -69.0276)
  line L609 (-148.3504, -72.4808) -> (-148.3855, -72.8823)
  line L610 (-77.4602, -68.5767) -> (-77.4602, -68.559)
  line L611 (-92.8836, -67.3531) -> (-92.8846, -67.1853)
  line L612 (-120.9345, -72.8083) -> (-120.8032, -72.878)
  line L613 (-115.0167, -69.5432) -> (-114.9978, -69.2913)
  line L614 (-169.0144, -78.3864) -> (-168.8644, -78.4586)
  line L615 (-89.5747, -78.1332) -> (-89.682, -78.0196)
  line L616 (-121.4576, -71.6475) -> (-121.4694, -71.7956)
  line L617 (-53.8827, -82.4721) -> (-53.7786, -82.603)
  line L618 (-115.6806, -75.595) -> (-115.7616, -75.4972)
  line L619 (-68.3883, -81.4192) -> (-68.4557, -81.3291)
  line L620 (-118.4636, -69.1947) -> (-118.4726, -69.384)
  line L621 (-77.5308, -80.931) -> (-77.4919, -80.7493)
  line L622 (-89.9704, -82.2161) -> (-90.0311, -82.05)
  line L623 (-56.1225, -68.7825) -> (-55.9677, -68.8427)
  line L624 (-119.5906, -65.5093) -> (-119.9188, -65.542)
  line L625 (-169.8348, -77.3883) -> (-169.7772, -77.5459)
  line L626 (-115.9387, -77.4488) -> (-115.8386, -77.3695)
  line L627 (-169.4097, -75.8909) -> (-169.5204, -75.9706)
  line L628 (-65.2174, -72.0012) -> (-65.2234, -72.2146)
  line L629 (-118.6897, -70.0123) -> (-118.7882, -70.1398)
  line L630 (-169.5204, -75.9706) -> (-169.6191, -76.0618)
  line L631 (-46.2553, -82.5297) -> (-46.2159, -82.4222)
  line L632 (-117.1313, -65.8656) -> (-117.2991, -65.7945)
  line L633 (-115.4725, -70.9992) -> (-115.3749, -70.8221)
  line L634 (-163.9927, -78.2379) -> (-163.882, -78.3083)
  line L635 (-115.5319, -76.9681) -> (-115.483, -76.8451)
  line L636 (-86.8066, -82.5231) -> (-86.9106, -82.6623)
  line L637 (-46.3632, -82.7285) -> (-46.3046, -82.632)
  line L638 (-77.0536, -75.9384) -> (-77.1657, -75.9096)
  line L639 (-123.2458, -69.3535) -> (-123.1293, -69.1355)
  line L640 (-116.4057, -77.6908) -> (-116.2806, -77.641)
  line L641 (-126.7473, -76.0244) -> (-126.6674, -76.2071)
  line L642 (-118.1807, -65.547) -> (-118.3631, -65.5198)
  line L643 (-126.5733, -76.3809) -> (-126.465, -76.546)
  line L644 (-118.3631, -65.5198) -> (-118.5467, -65.5002)
  line L645 (-86.7161, -80.6511) -> (-86.64, -80.809)
  line L646 (-116.2806, -77.641) -> (-116.1605, -77.5843)
  line L647 (-119.7714, -67.8329) -> (-119.5881, -67.881)
  line L648 (-83.5472, -77.0903) -> (-83.5412, -77.2401)
  line L649 (-126.2062, -76.8507) -> (-126.0559, -76.9907)
  line L650 (-123.1293, -69.1355) -> (-122.9886, -68.9274)
  line L651 (-98.4858, -73.0619) -> (-101.1722, -66.6714)
  line L652 (-78.8216, -82.0548) -> (-78.6478, -82.0202)
  line L653 (-126.1707, -65.5395) -> (-126.3132, -65.5816)
  line L654 (-156.201, -71.3588) -> (-156.4103, -71.3628)
  line L655 (-129.4881, -81.5151) -> (-129.5467, -81.4186)
  line L656 (-54.3315, -70.9062) -> (-54.2977, -71.0913)
  line L657 (-112.5222, -66.7004) -> (-112.5708, -66.858)
  line L658 (-126.3426, -76.7026) -> (-126.2062, -76.8507)
  line L659 (-123.1964, -78.0833) -> (-122.8727, -78.1301)
  line L660 (-116.5347, -77.734) -> (-116.4057, -77.6908)
  line L661 (-115.4247, -76.5699) -> (-115.4167, -76.4171)
  line L662 (-115.8386, -77.3695) -> (-115.747, -77.2821)
  line L663 (-121.4259, -71.5165) -> (-121.4576, -71.6475)
  line L664 (-135.6585, -71.8872) -> (-135.8284, -71.5777)
  line L665 (-119.5376, -70.6259) -> (-119.7376, -70.6965)
  line L666 (-135.54, -73.9208) -> (-135.4936, -73.7968)
  line L667 (-50.5439, -70.1959) -> (-50.6339, -69.8368)
  line L668 (-116.3294, -75.1745) -> (-116.4755, -75.1533)
  line L669 (-65.458, -67.7795) -> (-65.3418, -67.7972)
  line L670 (-72.7278, -66.0408) -> (-72.8225, -66.17)
  line L671 (-68.1943, -82.1936) -> (-68.1883, -82.0739)
  line L672 (-130.3974, -83.2377) -> (-130.2812, -83.22)
  line L673 (-125.8917, -77.1225) -> (-125.7138, -77.2464)
  line L674 (-116.8014, -77.8018) -> (-116.5347, -77.734)
  line L675 (-86.6995, -77.6175) -> (-86.7617, -77.7607)
  line L676 (-53.7786, -82.603) -> (-53.6624, -82.7225)
  line L677 (-141.7958, -65.6248) -> (-141.9397, -65.6991)
  line L678 (-129.6896, -82.9009) -> (-129.6141, -82.8178)
  line L679 (-117.6443, -65.6736) -> (-117.8209, -65.624)
  line L680 (-89.9976, -66.7159) -> (-89.961, -66.5581)
  line L681 (-115.483, -76.8451) -> (-115.447, -76.7125)
  line L682 (-112.0694, -66.0184) -> (-112.1863, -66.137)
  line L683 (-115.747, -77.2821) -> (-115.6648, -77.1863)
  line L684 (-122.8244, -68.7308) -> (-122.6372, -68.5476)
  line L685 (-115.4167, -76.4171) -> (-115.4217, -76.295)
  line L686 (-123.5073, -78.0302) -> (-123.1964, -78.0833)
  line L687 (-77.4602, -75.8859) -> (-77.4602, -68.5767)
  line L688 (-135.9986, -71.3165) -> (-136.1478, -71.1145)
  line L689 (-87.842, -65.5214) -> (-87.6422, -65.5656)
  line L690 (-126.465, -76.546) -> (-126.3426, -76.7026)
  line L691 (-126.0559, -76.9907) -> (-125.8917, -77.1225)
  line L692 (-120.2756, -73.0155) -> (-120.0568, -73.0282)
  line L693 (-126.0231, -65.5089) -> (-126.1707, -65.5395)
  line L694 (-72.2263, -65.6578) -> (-72.3691, -65.7333)
  line L695 (-125.317, -77.4711) -> (-125.0983, -77.5721)
  line L696 (-122.4745, -75.5935) -> (-122.6439, -75.5491)
  line L697 (-55.0598, -69.4503) -> (-54.9561, -69.5643)
  line L698 (-93.5202, -77.614) -> (-93.4808, -77.5065)
  line L699 (-159.6623, -76.9336) -> (-159.7115, -76.8314)
  line L700 (-123.4576, -71.6447) -> (-123.4576, -70.2886)
  line L701 (-56.9471, -65.4152) -> (-57.3582, -65.3964)
  line L702 (-127.0093, -66.0492) -> (-127.0901, -66.1588)
  line L703 (-46.4306, -81.3294) -> (-46.5062, -81.2463)
  line L704 (-93.7711, -76.3306) -> (-93.8542, -76.2551)
  line L705 (-115.2876, -70.6352) -> (-115.2109, -70.4382)
  line L706 (-93.4808, -77.5065) -> (-93.4519, -77.3943)
  line L707 (-50.4697, -70.5698) -> (-50.5439, -70.1959)
  line L708 (-111.4862, -65.6666) -> (-111.6483, -65.734)
  line L709 (-109.8263, -65.9506) -> (-109.9302, -65.8727)
  line L710 (-125.0983, -77.5721) -> (-124.8662, -77.6658)
  line L711 (-86.5793, -80.975) -> (-86.5348, -81.1482)
  line L712 (-79.5715, -82.0548) -> (-79.3885, -82.0756)
  line L713 (-125.7138, -77.2464) -> (-125.5222, -77.3626)
  line L714 (-161.5406, -66.0405) -> (-161.6481, -65.9247)
  line L715 (-46.2159, -82.4222) -> (-46.187, -82.31)
  line L716 (-83.5221, -76.8021) -> (-83.5412, -76.9402)
  line L717 (-87.7677, -79.7872) -> (-87.6017, -79.8479)
  line L718 (-142.0749, -65.7869) -> (-142.2007, -65.8871)
  line L719 (-86.5888, -77.145) -> (-86.6139, -77.3087)
  line L720 (-104.1537, -66.3521) -> (-104.1992, -66.4149)
  line L721 (-163.0667, -78.5355) -> (-162.9081, -78.5405)
  line L722 (-87.2947, -83.0114) -> (-87.4437, -83.1019)
  line L723 (-54.6852, -69.9478) -> (-54.6086, -70.0896)
  line L724 (-129.6141, -81.3285) -> (-129.6896, -81.2454)
  line L725 (-156.9307, -71.4261) -> (-157.0707, -71.4672)
  line L726 (-118.5467, -65.5002) -> (-118.7311, -65.4883)
  line L727 (-54.2064, -81.6625) -> (-54.1692, -81.8436)
  line L728 (-82.1648, -78.2274) -> (-81.9787, -78.2305)
  line L729 (-164.3546, -77.8655) -> (-164.2768, -77.9721)
  line L730 (-162.8379, -78.5345) -> (-162.72, -78.5529)
  line L731 (-65.8766, -67.6036) -> (-65.7801, -67.6622)
  line L732 (-54.7687, -69.813) -> (-54.6852, -69.9478)
  line L733 (-132.4933, -65.4916) -> (-132.6853, -65.4846)
  line L734 (-169.903, -76.7078) -> (-169.912, -76.8783)
  line L735 (-55.6766, -68.9828) -> (-55.5404, -69.0628)
  line L736 (-50.4116, -70.9586) -> (-50.4697, -70.5698)
  line L737 (-115.5025, -75.9293) -> (-115.551, -75.8125)
  line L738 (-164.3709, -66.1697) -> (-164.4525, -66.3121)
  line L739 (-116.2573, -71.8716) -> (-116.1043, -71.7474)
  line L740 (-140.8458, -65.5044) -> (-140.9924, -65.4901)
  line L741 (-112.3816, -66.403) -> (-112.459, -66.5484)
  line L742 (-169.7772, -76.2808) -> (-169.8348, -76.4096)
  line L743 (-47.0979, -80.9274) -> (-47.2141, -80.9097)
  line L744 (-66.2516, -66.076) -> (-66.3009, -66.1782)
  line L745 (-164.6445, -67.2203) -> (-164.6445, -69.8598)
  line L746 (-164.4525, -66.3121) -> (-164.5203, -66.4677)
  line L747 (-102.6019, -65.6294) -> (-102.7483, -65.6214)
  line L748 (-109.9302, -65.8727) -> (-110.0394, -65.803)
  line L749 (-54.0404, -66.0248) -> (-54.3644, -65.9031)
  line L750 (-95.8873, -75.988) -> (-92.9826, -67.8593)
  line L751 (-69.624, -67.2204) -> (-69.632, -67.0129)
  line L752 (-164.6365, -67.0127) -> (-164.6445, -67.2203)
  line L753 (-169.6191, -77.8372) -> (-169.5204, -77.9693)
  line L754 (-164.2768, -77.9721) -> (-164.1904, -78.0698)
  line L755 (-54.2524, -71.4835) -> (-54.241, -71.6908)
  line L756 (-115.9561, -75.3306) -> (-116.0697, -75.2646)
  line L757 (-161.8993, -65.7331) -> (-162.0421, -65.6576)
  line L758 (-122.1967, -68.2279) -> (-121.9446, -68.0949)
  line L759 (-123.6722, -67.5054) -> (-123.6866, -67.3062)
  line L760 (-103.7659, -65.9563) -> (-103.8578, -66.0282)
  line L761 (-60.9517, -70.0896) -> (-60.8751, -69.9478)
  line L762 (-86.5694, -76.8042) -> (-86.5744, -76.9765)
  line L763 (-116.6326, -75.1503) -> (-116.8006, -75.1659)
  line L764 (-115.551, -75.8125) -> (-115.6104, -75.7006)
  line L765 (-122.9443, -75.4272) -> (-123.0728, -75.3477)
  line L766 (-169.877, -76.5517) -> (-169.903, -76.7078)
  line L767 (-135.8284, -71.5777) -> (-135.9986, -71.3165)
  line L768 (-94.3095, -65.5904) -> (-94.4542, -65.5719)
  line L769 (-112.5744, -67.6917) -> (-112.5246, -67.8603)
  line L770 (-115.6104, -75.7006) -> (-115.6806, -75.595)
  line L771 (-155.841, -71.3363) -> (-155.9608, -71.3588)
  line L772 (-87.4437, -79.9239) -> (-87.2947, -80.0143)
  line L773 (-94.0408, -76.1291) -> (-94.1431, -76.0799)
  line L774 (-63.305, -65.7308) -> (-63.3951, -65.6634)
  line L775 (-141.8708, -77.2907) -> (-141.825, -77.4421)
  line L776 (-169.877, -77.2239) -> (-169.8348, -77.3883)
  line L777 (-162.1957, -65.5957) -> (-162.3596, -65.5474)
  line L778 (-93.4519, -77.3943) -> (-93.4342, -77.2781)
  line L779 (-79.7451, -82.0202) -> (-79.5715, -82.0548)
  line L780 (-115.9505, -66.6779) -> (-116.0791, -66.5536)
  line L781 (-124.5884, -65.7372) -> (-124.772, -65.6493)
  line L782 (-58.5464, -65.4115) -> (-58.9172, -65.4383)
  line L783 (-71.343, -83.2371) -> (-71.2172, -83.2441)
  line L784 (-169.8348, -76.4096) -> (-169.877, -76.5517)
  line L785 (-126.9296, -69.1468) -> (-126.9296, -74.973)
  line L786 (-162.9081, -78.5405) -> (-162.8379, -78.5345)
  line L787 (-129.353, -82.193) -> (-129.347, -82.0733)
  line L788 (-141.1327, -78.275) -> (-140.997, -78.3528)
  line L789 (-123.0728, -75.3477) -> (-123.185, -75.2544)
  line L790 (-60.3108, -65.654) -> (-60.6361, -65.7353)
  line L791 (-115.4648, -76.0496) -> (-115.5025, -75.9293)
  line L792 (-162.9082, -65.4849) -> (-163.1, -65.4919)
  line L793 (-121.9446, -68.0949) -> (-121.6721, -67.9822)
  line L794 (-63.895, -83.1446) -> (-63.6988, -83.1888)
  line L795 (-121.2699, -75.693) -> (-121.6987, -75.685)
  line L796 (-76.8438, -78.0852) -> (-76.7473, -78.0266)
  line L797 (-145.1341, -73.9113) -> (-145.0573, -73.5791)
  line L798 (-169.1558, -78.3005) -> (-169.0144, -78.3864)
  line L799 (-120.7434, -70.9215) -> (-120.8538, -70.9601)
  line L800 (-57.3582, -65.3964) -> (-57.7791, -65.3904)
  line L801 (-116.1941, -75.2121) -> (-116.3294, -75.1745)
  line L802 (-88.6697, -83.2833) -> (-88.8429, -83.2388)
  line L803 (-46.2159, -81.7259) -> (-46.2553, -81.6183)
  line L804 (-80.7403, -81.2552) -> (-80.6588, -81.3976)
  line L805 (-66.3403, -66.2857) -> (-66.3691, -66.3979)
  line L806 (-130.9496, -67.22) -> (-130.9576, -67.0124)
  line L807 (-162.7163, -65.4919) -> (-162.9082, -65.4849)
  line L808 (-101.4211, -66.2621) -> (-101.4961, -66.1748)
  line L809 (-139.075, -78.0114) -> (-138.937, -77.8736)
  line L810 (-165.4074, -78.3891) -> (-165.2902, -78.3193)